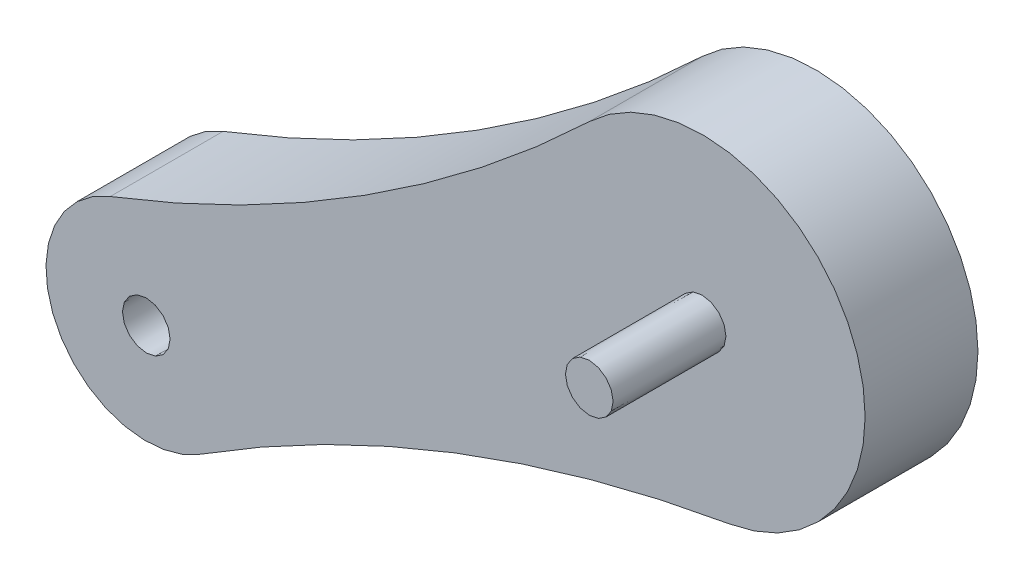
# Autodesk Inventor part: Нога
Saved by Autodesk Inventor 2026 (Build 300175000, 175)
## iProperties
Created: 2026-04-19
Part Number: Нога
Material: Типовые
Document SubType Name: Modeling
Designer: Artem Sannikov
Density: 1 g/cm^3
Appearance: По умолчанию
Author: Artem Sannikov
Autodesk Inventor part; units mm, degrees
ref_plane "YZ Plane" through (0, 0, 0) normal (1, 0, 0) x (0, 1, 0)
ref_plane "XZ Plane" through (0, 0, 0) normal (0, 1, 0) x (-1, 0, 0)
ref_plane "XY Plane" through (0, 0, 0) normal (0, 0, 1) x (1, 0, 0)
sketch "Эскиз1" plane through (0, 0, 0) normal (0, 0, 1) x (1, 0, 0)
  point P0 (0, 0)
sketch "Эскиз2" plane through (0, 0, 0) normal (0, 0, 1) x (1, 0, 0)
  circle A0 centre (0, 0) radius 9.5
  dimension "d0" = 19
  constraints: 1 centre point, 1 coincident
  measures "d0" diameter of A0
extrude "Выдавливание1" add sketch "Эскиз2" against normal blind 5
sketch "Эскиз3" plane through (0, 0, 0) normal (0, 0, 1) x (1, 0, 0)
  circle A0 centre (0, 0) radius 40
  circle A1 centre (0, 0) radius 9.5 projected
  line L0 (0, 0) -> (221.6445, 111.8073) construction
  arc A2 (-18.0154, 35.7134) -> (18.0154, -35.7134) centre (0, 0) ccw
  arc A3 (250.9196, 53.7731) -> (192.3695, 169.8415) centre (221.6445, 111.8073) ccw
  circle A4 centre (221.6445, 111.8073) radius 65
  circle A5 centre (330.0256, -518.949) radius 575
  circle A6 centre (-221.2225, 573.8341) radius 575
  circle A7 centre (221.6445, 111.8073) radius 10 projected
  point P0 (110.8223, 55.9037)
  point P1 (-14.3885, 37.3225)
  point P2 (21.4651, -33.7528)
  point P3 (232.652, 47.7461)
  point P4 (250.9196, 53.7731)
  point P5 (192.3695, 169.8415)
  point P6 (176.6659, 158.7319)
  dimension "d3" = 80
  dimension "d4" = 1150
  dimension "d10" = 65
  constraints: 6 centre point, 4 end point, 4 point on circle, 3 coincident, 2 concentric, 2 tangent, 1 midpoint, 1 symmetric about line, 1 other
  measures "d3" diameter of A0
  measures "d4" diameter of A5
  measures "d10" radius of A3
extrude "Выдавливание2" add sketch "Эскиз3" along normal blind 45 contours A0 | A6 A4 A5 A0 | A4 A3 | A7
sketch "Эскиз4" plane through (0, 0, 45) normal (0, 0, 1) x (1, 0, 0)
  point P0 (0, 0)
sketch "Эскиз5" plane through (0, 0, 45) normal (0, 0, 1) x (1, 0, 0)
  arc A0 (232.652, 47.7461) -> (176.6659, 158.7319) centre (221.6445, 111.8073) ccw projected
  circle A1 centre (221.6445, 111.8073) radius 9.5
  point P0 (0, 0)
  dimension "d7" = 19
  constraints: 1 centre point, 1 coincident
  measures "d7" diameter of A1
extrude "Выдавливание3" add sketch "Эскиз5" along normal blind 45
